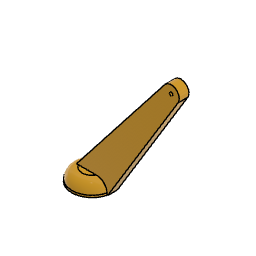
primerbrazo v8 (Autodesk Fusion 360 design; units mm, degrees)
Autodesk Fusion 360 part; units mm, degrees
sketch "Sketch1" plane through (0, 0, 0) normal (0, 0, 1) x (1, 0, 0)
  circle A0 centre (0, 0) radius 125
  dimension "d1" = 250
  constraint coincident A0.centre origin
  measures "d1" diameter of A0
extrude "Extrude1" add sketch "Sketch1" along normal blind 75
fillet "Fillet1" radius 62.5 1 edges at (-116.5409, -45.2019, 75)
sketch "Sketch2" plane through (0, 0, 0) normal (0, 0, -1) x (1, 0, 0)
  circle A0 centre (0, 0) radius 125
  circle A1 centre (0, 0) radius 25
  dimension "d6" = 50
  constraint coincident A0.centre A1.centre
  measures "d6" diameter of A1
extrude "Extrude2" cut sketch "Sketch2" against normal blind 25 contours A1
sketch "Sketch3" plane through (0, 0, 0) normal (0, 1, 0) x (1, 0, 0)
  line L0 (62.5, -75) -> (-62.5, -75)
  line L1 (-125, 0) -> (125, 0)
  line L2 (-125, 0) -> (478.3021, -770.2875)
  line L3 (125, 0) -> (560.3465, -713.412)
  arc A0 (478.3021, -770.2875) -> (560.3465, -713.412) centre (517.6658, -739.4572) ccw
  circle A1 centre (517.6658, -739.4572) radius 10
  dimension "d23" = 100
  dimension "d24" = 20
  constraint coincident L1.start L2.start
  constraint tangent L2 A0
  constraint coincident L1.end L3.start
  constraint tangent L3 A0
  constraint concentric A0 A1
  measures "d23" diameter of A0
  measures "d24" diameter of A1
extrude "Extrude6" add sketch "Sketch3" along normal blind 30 and the other way blind 30
sketch "Sketch5" plane through (0, 0, 0) normal (0, 0, -1) x (1, 0, 0)
  arc A0 (121.3466, 30) -> (-121.3466, 30) centre (0, 0) ccw
  line L0 (-121.3466, 30) -> (-125, 30)
  line L1 (-125, 30) -> (-125, 0)
  line L2 (-125, 0) -> (-125, -30)
  line L3 (-125, -30) -> (-121.3466, -30)
  arc A1 (-121.3466, -30) -> (121.3466, -30) centre (0, 0) ccw
  line L4 (121.3466, -30) -> (125, -30)
  line L5 (125, -30) -> (125, 30)
  line L6 (125, 30) -> (121.3466, 30)
  circle A2 centre (0, 0) radius 25
  dimension "d29" = 50
  constraint coincident A0.centre A1.centre
  measures "d29" diameter of A2
extrude "Extrude7" cut sketch "Sketch5" against normal blind 30 contours A2
scale "Scale1" factor 2.5 about (0, 0, 0) bodies 1
